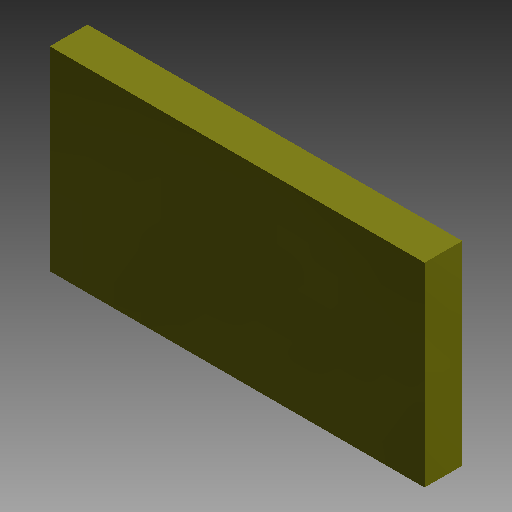
# Autodesk Inventor part: 0.6r
Saved by Autodesk Inventor 2018.2 (Build 222227000, 227)
## iProperties
Part Number: 0.6r
Material: Generic
Document SubType Name: Modeling
Designer: autocad
Appearance: 2512R-0.55, 0.6r
Author: autocad
Autodesk Inventor part; units mm, degrees
ref_plane "YZ Plane" through (0, 0, 0) normal (1, 0, 0) x (0, 1, 0)
ref_plane "XZ Plane" through (0, 0, 0) normal (0, 1, 0) x (-1, 0, 0)
ref_plane "XY Plane" through (0, 0, 0) normal (0, 0, 1) x (1, 0, 0)
sketch "2512R-0.55, 0.6r_315" plane through (0, 0, 0) normal (0, 0, 1) x (1, 0, 0)
  line L0 (-3.225, 1.675) -> (3.225, 1.675)
  line L1 (3.225, 1.675) -> (3.225, -1.675)
  line L2 (3.225, -1.675) -> (-3.225, -1.675)
  line L3 (-3.225, -1.675) -> (-3.225, 1.675)
  constraints: 8 end point
extrude "Extrusion1" add sketch "2512R-0.55, 0.6r_315" along normal blind 0.65
body "Solid1"
